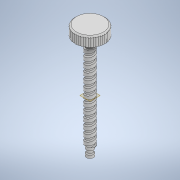
# Autodesk Inventor part: lead_screw
Saved by Autodesk Inventor 2021 (Build 250183000, 183)
## iProperties
Created: 2020-07-09
Part Number: lead_screw
Material: Generic
Document SubType Name: Modeling
Designer: Daniel
Density: 1 g/cm^3
Appearance: Default
Author: Daniel
Autodesk Inventor part; units mm, degrees
ref_plane "YZ Plane" through (0, 0, 0) normal (1, 0, 0) x (0, 1, 0)
ref_plane "XZ Plane" through (0, 0, 0) normal (0, 1, 0) x (-1, 0, 0)
ref_plane "XY Plane" through (0, 0, 0) normal (0, 0, 1) x (1, 0, 0)
sketch "Sketch1" plane through (0, 0, 0) normal (0, 1, 0) x (-1, 0, 0)
  circle A0 centre (0, 0) radius 4.95
  dimension "d0" = 9.9
  constraints: 1 centre point, 1 coincident
  measures "d0" diameter of A0
extrude "Extrusion1" add sketch "Sketch1" along normal blind 90
sketch "Sketch2" plane through (0, 0, 0) normal (0, 0, 1) x (-1, 0, 0)
  line L0 (4.95, 0) -> (4.95, 1.5)
  line L1 (4.95, 1.5) -> (3.651, 0.75) construction
  line L2 (4.95, 0) -> (3.651, 0.75)
  line L3 (-4.95, 0) -> (4.95, 0) construction
  line L4 (4.95, 0) -> (4.95, -90) projected
  line L5 (-4.95, -90) -> (-4.95, 0) projected
  line L6 (4.95, -90) -> (-4.95, -90) projected
  line L7 (4.95, 3.5) -> (3.651, 2.75)
  line L8 (3.651, 2.75) -> (3.651, 0.75)
  line L9 (4.95, 3.5) -> (4.95, 1.5)
  line L10 (-4.95, 0) -> (4.95, 0) projected
  point P0 (0, 0)
  dimension "d3" = 1.5
  dimension "d4" = 60
  dimension "d19" = 0
  dimension "d65" = 2
  constraints: 12 end point, 2 vertical, 1 collinear, 1 equal length, 1 parallel, 1 point on line
  measures "d3" distance of L0.start L0.end
  measures "d4" angle of L2 L1
  measures "d19" distance between parallel lines of L4 L0
  measures "d65" distance of L7.start L0.end
coil "Coil1" sketch "Sketch2" operation cut axis through (0, -10, 0) along (0, 1, 0) pitch 7 turns 13.857143 hand right contours L2 L8 L7 L9 L0
ref_plane "Work Plane1" through (0, 45, 0) normal (0, 1, 0) x (1, 0, 0)
sketch "Sketch8" plane through (0, 0, 0) normal (1, 0, 0) x (0, 1, 0)
  line L0 (90, 0) -> (100, 0)
  line L1 (100, 0) -> (100, -3.65)
  line L2 (100, -3.65) -> (90, -3.65)
  line L3 (90, -3.65) -> (90, 0)
  line L4 (92.9, -3.65) -> (97.1, -3.65)
  line L5 (97.1, -3.65) -> (97.1, -2.65)
  line L6 (97.1, -2.65) -> (92.9, -2.65)
  line L7 (92.9, -2.65) -> (92.9, -3.65)
  line L8 (90, -0.8124) -> (90, -0.8124) projected
  point P0 (0, 0)
  dimension "d50" = 10
  dimension "d51" = 3.65
  dimension "d52" = 4.2
  dimension "d53" = 2.9
  dimension "d54" = 1
  constraints: 16 end point, 4 parallel, 2 horizontal, 2 perpendicular, 2 point on line, 1 collinear
  measures "d50" distance of L1.end L2.end
  measures "d51" distance of L0.end L1.end
  measures "d52" distance of L5.end L6.end
  measures "d53" distance between parallel lines of L3 L7
  measures "d54" distance of L4.end L5.end
revolve "Revolution2" add sketch "Sketch8" angle 360 about axis through (0, 90, 0) along (0, 1, 0) contours L0 L1 L2 L5 L6 L7 L3
mirror "Mirror1" about plane through (0, 45, 0) normal (0, 1, 0) of "Revolution2"
sketch "Sketch7" plane through (0, 100, 0) normal (0, 1, 0) x (1, 0, 0)
  circle A0 centre (0, 0) radius 15
  circle A1 centre (0, -14.5) radius 1.25
  circle A2 centre (1.8173, -14.3857) radius 1.25
  circle A3 centre (3.606, -14.0445) radius 1.25
  circle A4 centre (5.3378, -13.4818) radius 1.25
  circle A5 centre (6.9854, -12.7064) radius 1.25
  circle A6 centre (8.5229, -11.7307) radius 1.25
  circle A7 centre (9.9259, -10.57) radius 1.25
  circle A8 centre (11.1724, -9.2426) radius 1.25
  circle A9 centre (12.2428, -7.7695) radius 1.25
  circle A10 centre (13.12, -6.1738) radius 1.25
  circle A11 centre (13.7903, -4.4807) radius 1.25
  circle A12 centre (14.2432, -2.717) radius 1.25
  circle A13 centre (14.4714, -0.9105) radius 1.25
  circle A14 centre (14.4714, 0.9105) radius 1.25
  circle A15 centre (14.2432, 2.717) radius 1.25
  circle A16 centre (13.7903, 4.4807) radius 1.25
  circle A17 centre (13.12, 6.1738) radius 1.25
  circle A18 centre (12.2428, 7.7695) radius 1.25
  circle A19 centre (11.1724, 9.2426) radius 1.25
  circle A20 centre (9.9259, 10.57) radius 1.25
  circle A21 centre (8.5229, 11.7307) radius 1.25
  circle A22 centre (6.9854, 12.7064) radius 1.25
  circle A23 centre (5.3378, 13.4818) radius 1.25
  circle A24 centre (3.606, 14.0445) radius 1.25
  circle A25 centre (1.8173, 14.3857) radius 1.25
  circle A26 centre (0, 14.5) radius 1.25
  circle A27 centre (-1.8173, 14.3857) radius 1.25
  circle A28 centre (-3.606, 14.0445) radius 1.25
  circle A29 centre (-5.3378, 13.4818) radius 1.25
  circle A30 centre (-6.9854, 12.7064) radius 1.25
  circle A31 centre (-8.5229, 11.7307) radius 1.25
  circle A32 centre (-9.9259, 10.57) radius 1.25
  circle A33 centre (-11.1724, 9.2426) radius 1.25
  circle A34 centre (-12.2428, 7.7695) radius 1.25
  circle A35 centre (-13.12, 6.1738) radius 1.25
  circle A36 centre (-13.7903, 4.4807) radius 1.25
  circle A37 centre (-14.2432, 2.717) radius 1.25
  circle A38 centre (-14.4714, 0.9105) radius 1.25
  circle A39 centre (-14.4714, -0.9105) radius 1.25
  circle A40 centre (-14.2432, -2.717) radius 1.25
  circle A41 centre (-13.7903, -4.4807) radius 1.25
  circle A42 centre (-13.12, -6.1738) radius 1.25
  circle A43 centre (-12.2428, -7.7695) radius 1.25
  circle A44 centre (-11.1724, -9.2426) radius 1.25
  circle A45 centre (-9.9259, -10.57) radius 1.25
  circle A46 centre (-8.5229, -11.7307) radius 1.25
  circle A47 centre (-6.9854, -12.7064) radius 1.25
  circle A48 centre (-5.3378, -13.4818) radius 1.25
  circle A49 centre (-3.606, -14.0445) radius 1.25
  circle A50 centre (-1.8173, -14.3857) radius 1.25
  point P0 (0.9624, -15.2976)
  point P1 (2.8722, -15.0564)
  point P2 (4.7366, -14.5777)
  point P3 (6.5263, -13.8691)
  point P4 (8.2131, -12.9417)
  point P5 (8.6785, -10.4905)
  point P6 (11.1735, -10.4926)
  point P7 (12.4005, -9.0095)
  point P8 (13.4319, -7.3843)
  point P9 (14.2515, -5.6426)
  point P10 (14.8463, -3.8119)
  point P11 (15.207, -1.9211)
  point P12 (15.3279, 0)
  point P13 (15.207, 1.9211)
  point P14 (14.8463, 3.8119)
  point P15 (14.2515, 5.6426)
  point P16 (13.4319, 7.3843)
  point P17 (12.4005, 9.0095)
  point P18 (11.1735, 10.4926)
  point P19 (9.7704, 11.8103)
  point P20 (8.2131, 12.9417)
  point P21 (6.5263, 13.8691)
  point P22 (4.7366, 14.5777)
  point P23 (2.8722, 15.0564)
  point P24 (0.9624, 15.2976)
  point P25 (-0.9624, 15.2976)
  point P26 (-2.8722, 15.0564)
  point P27 (-4.7366, 14.5777)
  point P28 (-6.5263, 13.8691)
  point P29 (-8.2131, 12.9417)
  point P30 (-9.7704, 11.8103)
  point P31 (-11.1735, 10.4926)
  point P32 (-12.4005, 9.0095)
  point P33 (-13.4319, 7.3843)
  point P34 (-14.2515, 5.6426)
  point P35 (-14.8463, 3.8119)
  point P36 (-15.207, 1.9211)
  point P37 (-15.3279, 0)
  point P38 (-15.207, -1.9211)
  point P39 (-14.8463, -3.8119)
  point P40 (-14.2515, -5.6426)
  point P41 (-13.4319, -7.3843)
  point P42 (-12.4005, -9.0095)
  point P43 (-11.1735, -10.4926)
  point P44 (-9.7704, -11.8103)
  point P45 (-8.2131, -12.9417)
  point P46 (-6.5263, -13.8691)
  point P47 (-4.7366, -14.5777)
  point P48 (-2.8722, -15.0564)
  point P49 (-0.9624, -15.2976)
  point P50 (-2.5512, -13.3738)
  point P51 (-0.8549, -13.588)
  point P52 (0.8549, -13.588)
  point P53 (2.5512, -13.3738)
  point P54 (4.2072, -12.9485)
  point P55 (5.7969, -12.3191)
  point P56 (7.2952, -11.4954)
  point P57 (9.9248, -9.32)
  point P58 (11.0147, -8.0026)
  point P59 (11.9308, -6.559)
  point P60 (12.6588, -5.012)
  point P61 (13.1872, -3.3859)
  point P62 (13.5075, -1.7064)
  point P63 (13.6149, 0)
  point P64 (13.5075, 1.7064)
  point P65 (13.1872, 3.3859)
  point P66 (12.6588, 5.012)
  point P67 (11.9308, 6.559)
  point P68 (11.0147, 8.0026)
  point P69 (9.9248, 9.32)
  point P70 (8.6785, 10.4905)
  point P71 (7.2952, 11.4954)
  point P72 (5.7969, 12.3191)
  point P73 (4.2072, 12.9485)
  point P74 (2.5512, 13.3738)
  point P75 (0.8549, 13.588)
  point P76 (-0.8549, 13.588)
  point P77 (-2.5512, 13.3738)
  point P78 (-4.2072, 12.9485)
  point P79 (-5.7969, 12.3191)
  point P80 (-7.2952, 11.4954)
  point P81 (-8.6785, 10.4905)
  point P82 (-9.9248, 9.32)
  point P83 (-11.0147, 8.0026)
  point P84 (-11.9308, 6.559)
  point P85 (-12.6588, 5.012)
  point P86 (-13.1872, 3.3859)
  point P87 (-13.5075, 1.7064)
  point P88 (-13.6149, 0)
  point P89 (-13.5075, -1.7064)
  point P90 (-13.1872, -3.3859)
  point P91 (-12.6588, -5.012)
  point P92 (-11.9308, -6.559)
  point P93 (-11.0147, -8.0026)
  point P94 (-9.9248, -9.32)
  point P95 (-8.6785, -10.4905)
  point P96 (-7.2952, -11.4954)
  point P97 (-5.7969, -12.3191)
  point P98 (-4.2072, -12.9485)
  point P99 (9.7704, -11.8103)
  dimension "d39" = 2.5
  dimension "d40" = 30
  dimension "d41" = 14.5
  dimension "d44" = 360
  constraints: 51 centre point, 1 coincident, 101 other
  measures "d39" diameter of A1
  measures "d40" diameter of A0
  measures "d41" distance of A0.centre A1.centre
extrude "Extrusion5" add sketch "Sketch7" along normal blind 10
fillet "Fillet1" radius 2 1 edges at (0, 100, 3.65)
chamfer "Chamfer4" distance 1 angle 45 2 edges at (0, 92.9, 2.65) (0, -7.1, 2.65)
sketch "Sketch9" plane through (0, 0, 0) normal (1, 0, 0) x (0, 1, 0)
  line L0 (108, 16.15) -> (112.6492, 11.5008)
  line L1 (108, 16.15) -> (114.5749, 16.15) construction
  line L2 (112.6492, 11.5008) -> (112.6492, 16.15)
  line L3 (100, 15.0564) -> (110, 15.0564) projected
  line L4 (112.6492, 16.15) -> (108, 16.15)
  line L5 (97.1, 3.65) -> (97.1, -3.65) projected
  line L6 (97.1, 0) -> (124.7436, 0)
  line L7 (98, -3.65) -> (98, 3.65) projected
  point P0 (0, 0)
  dimension "d63" = 45
  dimension "d66" = 10
  dimension "d67" = 12.5
  constraints: 10 end point, 2 horizontal, 2 perpendicular, 1 equal length, 1 midpoint
  measures "d63" angle of L0 L1
  measures "d66" distance from line of L7 L0.start
  measures "d67" vertical distance of L7.end L0.start
revolve "Revolution3" cut sketch "Sketch9" angle 360 about axis through (0, 97.1, 0) along (0, 1, 0)
equation "\"d1\" = length"
equation "\"d8\" = pitch"
equation "\"d9\" = pitch + length"
equation "\"pitch\" = 7"
equation "\"length\" = 90"
body "Solid1"
